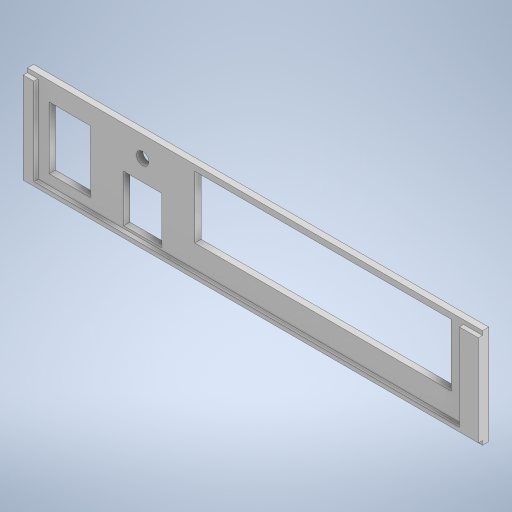
# Autodesk Inventor part: front_panel
Saved by Autodesk Inventor 2023 (Build 270158000, 158)
## iProperties
Created: 2023-05-16
Part Number: front_panel
Material: Generic
Document SubType Name: Modeling
Designer: mark
Density: 1 g/cm^3
Appearance: Default
Author: mark
Autodesk Inventor part; units mm, degrees
ref_plane "YZ Plane" through (0, 0, 0) normal (1, 0, 0) x (0, 1, 0)
ref_plane "XZ Plane" through (0, 0, 0) normal (0, 1, 0) x (-1, 0, 0)
sketch "Sketch1" plane through (0, 0, 0) normal (0, 1, 0) x (-1, 0, 0)
  line L0 (60, -40) -> (-60, -40)
  line L1 (-65, -35) -> (-65, 35)
  line L2 (-60, 40) -> (60, 40)
  line L3 (65, 35) -> (65, -35)
  arc A0 (60, -40) -> (65, -35) centre (60, -35) ccw
  arc A1 (-65, -35) -> (-60, -40) centre (-60, -35) ccw
  arc A2 (-60, 40) -> (-65, 35) centre (-60, 35) ccw
  arc A3 (65, 35) -> (60, 40) centre (60, 35) ccw
  line L4 (60, -37.5) -> (-60, -37.5)
  line L5 (-62.5, -35) -> (-62.5, 35)
  line L6 (-60, 37.5) -> (60, 37.5)
  line L7 (62.5, 35) -> (62.5, -35)
  arc A4 (62.5, 35) -> (60, 37.5) centre (60, 35) ccw
  arc A5 (60, -37.5) -> (62.5, -35) centre (60, -35) ccw
  arc A6 (-62.5, -35) -> (-60, -37.5) centre (-60, -35) ccw
  arc A7 (-60, 37.5) -> (-62.5, 35) centre (-60, 35) ccw
  point P0 (0, 0)
  point P1 (-65, 40)
  point P2 (-65, -40)
  point P3 (65, 40)
  dimension "d0" = 130
  dimension "d1" = 80
  dimension "d2" = 5
  dimension "d3" = 2.5
  dimension "d4" = 2.5
  dimension "d5" = 2.5
  dimension "d6" = 2.5
  dimension "d7" = 2.5
  dimension "d32" = 65
  dimension "d33" = 40
  constraints: 16 end point, 16 point on circle, 16 tangent, 8 centre point, 6 equal radius, 6 point on line, 4 parallel, 2 horizontal, 2 perpendicular
  measures "d0" distance of point (-65, 40) point (65, 40)
  measures "d1" distance of point (-65, -40) point (-65, 40)
  measures "d2" radius of A0
  measures "d3" distance between parallel lines of L0 L4
  measures "d4" distance between parallel lines of L3 L7
  measures "d5" distance between parallel lines of L2 L6
  measures "d6" distance between parallel lines of L1 L5
  measures "d7" radius of A4
  measures "d32" distance from line of point (0, 0) L3
  measures "d33" distance from line of L2 point (0, 0)
extrude "Extrusion1" add sketch "Sketch1" along normal blind 24
sketch "Sketch2" plane through (0, 24, 0) normal (0, 1, 0) x (1, 0, 0)
  line L0 (-60, -38.5) -> (60, -38.5)
  line L1 (63.5, -35) -> (63.5, 35)
  line L2 (60, 38.5) -> (-60, 38.5)
  line L3 (-63.5, 35) -> (-63.5, -35)
  line L4 (-60, 37.5) -> (60, 37.5) projected
  line L5 (62.5, 35) -> (62.5, -35) projected
  line L6 (60, -37.5) -> (-60, -37.5) projected
  line L7 (-62.5, -35) -> (-62.5, 35) projected
  arc A0 (-63.5, -35) -> (-60, -38.5) centre (-60, -35) ccw
  arc A1 (-60, 38.5) -> (-63.5, 35) centre (-60, 35) ccw
  arc A2 (63.5, 35) -> (60, 38.5) centre (60, 35) ccw
  arc A3 (60, -38.5) -> (63.5, -35) centre (60, -35) ccw
  point P0 (0, 0)
  dimension "d10" = 1
  dimension "d11" = 1
  dimension "d12" = 1
  dimension "d13" = 1
  dimension "d14" = 3.5
  constraints: 8 end point, 8 point on circle, 8 tangent, 4 centre point, 3 equal radius, 2 parallel, 1 horizontal, 1 perpendicular
  measures "d10" distance between parallel lines of L4 L2
  measures "d11" distance between parallel lines of L1 L5
  measures "d12" distance between parallel lines of L6 L0
  measures "d13" distance between parallel lines of L7 L3
  measures "d14" radius of A0
extrude "Extrusion2" cut sketch "Sketch2" against normal blind 1
ref_plane "Work Plane1" through (0, 12, 0) normal (0, 1, 0) x (1, 0, 0)
mirror "Mirror1" about plane through (0, 12, 0) normal (0, 1, 0) of "Extrusion2"
sketch "Sketch3" plane through (0, 23, 0) normal (0, 1, 0) x (1, 0, 0)
  line L0 (-56.5, 37.5) -> (-62.5, 37.5)
  line L1 (-62.5, 37.5) -> (-62.5, 31.5)
  line L2 (-62.5, 31.5) -> (-56.5, 31.5)
  line L3 (-56.5, 31.5) -> (-56.5, 37.5)
  line L4 (60, 37.5) -> (-60, 37.5) projected
  line L5 (-62.5, 35) -> (-62.5, -35) projected
  circle A0 centre (-60, 35) radius 2.4
  arc A1 (-60, 37.5) -> (-62.5, 35) centre (-60, 35) ccw projected
  point P0 (0, 0)
  dimension "d18" = 6
  dimension "d19" = 6
  dimension "d20" = 4.8
  constraints: 10 end point, 2 collinear, 2 parallel, 1 centre point, 1 concentric, 1 horizontal, 1 perpendicular
  measures "d18" distance of L2.end L1.end
  measures "d19" distance of L1.end L0.end
  measures "d20" diameter of A0
extrude "Extrusion3" add sketch "Sketch3" against normal up to surface (22 mm away)
fillet "Fillet2" radius 3.5 1 edges at (-56.5, 12, -31.5)
mirror "Mirror2" about plane through (0, 0, 0) normal (0, 0, 1) of "Extrusion3", "Fillet2"
mirror "Mirror3" about plane through (0, 0, 0) normal (1, 0, 0) of "Fillet2", "Extrusion3", "Mirror2"
sketch "Sketch7" plane through (60, 0, -40) normal (0, 0, -1) x (-1, 0, 0)
  line L0 (13, 22.6) -> (75, 22.6)
  line L1 (75, 22.6) -> (75, 7.6)
  line L2 (75, 7.6) -> (13, 7.6)
  line L3 (13, 7.6) -> (13, 22.6)
  line L4 (-5, 0) -> (-5, 24) projected
  line L5 (0, 0) -> (120, 0) projected
  point P0 (60, 0)
  dimension "d35" = 62
  dimension "d36" = 15
  dimension "d37" = 18
  dimension "d38" = 7.6
  constraints: 8 end point, 2 parallel, 1 horizontal, 1 perpendicular
  measures "d35" distance of L1.end L2.end
  measures "d36" distance of L0.end L1.end
  measures "d37" distance between parallel lines of L3 L4
  measures "d38" distance between parallel lines of L5 L2
extrude "Extrusion4" cut sketch "Sketch7" against normal blind 24
sketch "Sketch8" plane through (-56.5, 1, -37.5) normal (0, 0, 1) x (1, 0, 0)
  line L0 (-3.5, 22) -> (116.5, 22) projected
  line L1 (3.6019, 22) -> (106.4534, 22)
  line L2 (106.4534, 22) -> (106.4534, 1)
  line L3 (106.4534, 1) -> (3.6019, 1)
  line L4 (3.6019, 1) -> (3.6019, 22)
  point P0 (56.5, -1)
  dimension "d43" = 21
  constraints: 8 end point, 2 parallel, 1 horizontal, 1 perpendicular, 1 point on line
  measures "d43" distance between parallel lines of L3 L0
extrude "Extrusion5" cut sketch "Sketch8" against normal blind 1
sketch "Sketch9" plane through (60, 0, -40) normal (0, 0, -1) x (-1, 0, 0)
  line L0 (83, 14) -> (92.2, 14)
  line L1 (92.2, 14) -> (92.2, 2.6)
  line L2 (92.2, 2.6) -> (83, 2.6)
  line L3 (83, 2.6) -> (83, 14)
  line L4 (75, 22.6) -> (75, 7.6) projected
  line L5 (100.2, 4.5) -> (110.2, 4.5)
  line L6 (110.2, 4.5) -> (110.2, 19.5)
  line L7 (110.2, 19.5) -> (100.2, 19.5)
  line L8 (100.2, 19.5) -> (100.2, 4.5)
  circle A0 centre (87.6, 19) radius 1.5
  line L9 (10.0466, 2) -> (112.8981, 2) projected
  line L10 (0, 24) -> (120, 24) projected
  point P0 (60, 0)
  point P1 (83, 8.3)
  dimension "d44" = 8
  dimension "d45" = 9.2
  dimension "d46" = 11.4
  dimension "d47" = 10
  dimension "d48" = 15
  dimension "d49" = 8
  dimension "d50" = 3
  dimension "d51" = 5
  dimension "d54" = 0.6
  dimension "d55" = 4.5
  constraints: 16 end point, 4 parallel, 2 horizontal, 2 perpendicular, 1 centre point, 1 midpoint
  measures "d44" distance from line of L4 point (83, 8.3)
  measures "d45" distance of L0.start L0.end
  measures "d46" distance of L2.end L0.start
  measures "d47" distance of L7.end L6.end
  measures "d48" distance of L6.end L5.end
  measures "d49" distance between parallel lines of L1 L8
  measures "d50" diameter of A0
  measures "d51" distance from line of L0 A0.centre
  measures "d54" distance between parallel lines of L9 L2
  measures "d55" distance between parallel lines of L10 L7
extrude "Extrusion6" cut sketch "Sketch9" against normal blind 2
sketch "Sketch10" plane through (0, 24, 0) normal (0, 1, 0) x (1, 0, 0)
  line L0 (-65.5813, 44.518) -> (-55.4636, 44.518)
  line L1 (-55.4636, 44.518) -> (-55.4636, 27.5938)
  line L2 (-55.4636, 27.5938) -> (54.5438, 27.5938)
  line L3 (54.5438, 27.5938) -> (54.5438, 46.5416)
  line L4 (54.5438, 46.5416) -> (69.4444, 46.5416)
  line L5 (69.4444, 46.5416) -> (73.6755, -45.2538)
  line L6 (73.6755, -45.2538) -> (-73.3076, -45.2538)
  line L7 (-73.3076, -45.2538) -> (-65.5813, 44.518)
  point P0 (0, 0)
  constraints: 16 end point, 4 perpendicular, 1 horizontal, 1 parallel
extrude "Extrusion7" cut sketch "Sketch10" against normal through all
equation "\"d4\" = d3"
equation "\"d5\" = d3"
equation "\"d6\" = d3"
equation "\"d32\" = 0.5 * d0"
equation "\"d33\" = 0.5 * d1"
equation "\"d11\" = d10"
equation "\"d12\" = d10"
equation "\"d13\" = d10"
body "Solid1"
